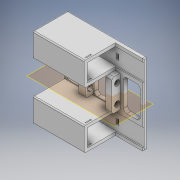
# Autodesk Inventor part: base_s
Saved by Autodesk Inventor 2020 (Build 240168000, 168)
## iProperties
Created: 2020-01-10
Part Number: base_s
Material: Generic
Document SubType Name: Modeling
Designer: Darien
Density: 1 g/cm^3
Appearance: Default
Author: Darien
Autodesk Inventor part; units mm, degrees
ref_plane "YZ Plane" through (0, 0, 0) normal (1, 0, 0) x (0, 1, 0)
ref_plane "XZ Plane" through (0, 0, 0) normal (0, 1, 0) x (-1, 0, 0)
sketch "Sketch1" plane through (0, 0, 0) normal (0, 0, 1) x (1, 0, 0)
  line L0 (-38.5, 45) -> (38.5, 45)
  line L1 (38.5, 45) -> (38.5, -45)
  line L2 (38.5, -45) -> (-38.5, -45)
  line L3 (-38.5, -45) -> (-38.5, 45)
  line L4 (-38.5, 45) -> (38.5, -45) construction
  line L5 (38.5, 45) -> (-38.5, -45) construction
  point P0 (0, 0)
  dimension "d0" = 90
  dimension "d1" = 77
  constraints: 12 end point, 2 midpoint, 2 parallel, 1 horizontal, 1 perpendicular
  measures "d0" distance of L1.end L0.end
  measures "d1" distance of L0.end L0.start
extrude "Extrusion1" add sketch "Sketch1" along normal blind 4
fillet "Fillet1" radius 4 4 edges at (-38.5, 45, 2) (-38.5, -45, 2) (38.5, 45, 2) (38.5, -45, 2)
sketch "Sketch15" plane through (0, 0, 4) normal (0, 0, 1) x (1, 0, 0)
  line L0 (34.5, 45) -> (-34.5, 45) construction
  line L1 (0, 45) -> (0, -45) construction
  line L2 (-34.5, -45) -> (34.5, -45) construction
  line L3 (-16, 15.4) -> (-10, 15.4)
  line L4 (-10, 15.4) -> (-10, -15)
  line L5 (-10, -15) -> (-16, -15)
  line L6 (-16, -15) -> (-16, 15.4)
  line L7 (-16, 15.4) -> (-10, -15) construction
  line L8 (-10, 15.4) -> (-16, -15) construction
  line L9 (16, 15.4) -> (10, 15.4)
  line L10 (10, 15.4) -> (10, -15)
  line L11 (10, -15) -> (16, -15)
  line L12 (16, -15) -> (16, 15.4)
  point P0 (-13, 0.2)
  dimension "d83" = 6
  dimension "d84" = 30.4
  dimension "d85" = 30
  dimension "d86" = 10
  constraints: 22 end point, 4 midpoint, 4 symmetric about line, 2 parallel, 1 horizontal, 1 perpendicular
  measures "d83" distance of L3.start L3.end
  measures "d84" distance of L5.end L3.start
  measures "d85" distance between parallel lines of L2 L5
  measures "d86" distance between parallel lines of L1 L4
extrude "Extrusion13" add sketch "Sketch15" along normal blind 7.8
sketch "Sketch16" plane through (16, -15.2, 4) normal (1, 0, 0) x (0, 0, -1)
  circle A0 centre (-2.75, 24.05) radius 2.65
  line L0 (-7.8, 0) -> (-7.8, 30.4) projected
  line L1 (0, 30.4) -> (-7.8, 30.4) projected
  line L2 (-7.8, 40.4) -> (-7.8, -10) construction
  line L3 (-7.8, 15.2) -> (0, 15.2) construction
  line L4 (0, -25.8) -> (0, 56.2) construction
  circle A1 centre (-2.75, 6.35) radius 2.65
  point P0 (4, 15.2)
  dimension "d62" = 5.05
  dimension "d63" = 6.35
  dimension "d64" = 5.3
  constraints: 2 centre point, 2 end point, 2 midpoint, 1 symmetric about line, 1 other
  measures "d62" distance from line of L0 A0.centre
  measures "d63" distance from line of L1 A0.centre
  measures "d64" diameter of A0
extrude "Extrusion14" cut sketch "Sketch16" against normal up to surface (32 mm away)
ref_plane "Work Plane2" through (17.25, -10.5, 0) normal (-1, 0, 0) x (0, 0, 1)
sketch "Sketch18" plane through (0, 0, 11.8) normal (0, 0, 1) x (1, 0, 0)
  line L0 (38.5, -41) -> (38.5, 41) projected
  line L1 (-38.5, -38.75) -> (38.5, -38.75)
  line L2 (38.5, -38.75) -> (38.5, 38.75)
  line L3 (38.5, 38.75) -> (-38.5, 38.75)
  line L4 (-38.5, 38.75) -> (-38.5, -38.75)
  line L5 (-38.5, -38.75) -> (38.5, 38.75) construction
  line L6 (38.5, -38.75) -> (-38.5, 38.75) construction
  line L7 (-38.5, -45.0251) -> (38.5, -45.0251)
  line L8 (38.5, -45.0251) -> (38.5, 45.0251)
  line L9 (38.5, 45.0251) -> (-38.5, 45.0251)
  line L10 (-38.5, 45.0251) -> (-38.5, -45.0251)
  line L11 (-38.5, -45.0251) -> (38.5, 45.0251) construction
  line L12 (38.5, -45.0251) -> (-38.5, 45.0251) construction
  point P0 (0, 0)
  point P1 (-38.5, 38.75)
  point P2 (-38.5, -38.75)
  dimension "d76" = 77.5
  constraints: 24 end point, 4 midpoint, 4 parallel, 2 horizontal, 2 perpendicular, 2 point on line
  measures "d76" distance between parallel lines of L3 L1
extrude "Extrusion16" cut sketch "Sketch18" against normal through all contours L8 L7 L10 L1 L0 | L3 L10 L9 L8 L0
sketch "Sketch19" plane through (10, -15, 4) normal (-1, 0, 0) x (0, 0, 1)
  circle A0 centre (2.75, 23.85) radius 2.65 projected
  circle A1 centre (2.75, 23.85) radius 3.2
  line L0 (0, 0) -> (0, 30.4) projected
  line L1 (0, 22.2137) -> (-0.0421, 25.4134)
  line L2 (-0.0421, 25.4134) -> (2.7079, 27.0497)
  line L3 (2.7079, 27.0497) -> (5.5, 25.4863)
  line L4 (5.5, 25.4863) -> (5.5421, 22.2866)
  line L5 (5.5421, 22.2866) -> (2.7921, 20.6503)
  line L6 (2.7921, 20.6503) -> (0, 22.2137)
  line L7 (0, 15.2) -> (7.8, 15.2)
  line L8 (7.8, 30.4) -> (7.8, 0) projected
  circle A2 centre (2.75, 6.55) radius 2.65
  circle A3 centre (2.75, 6.55) radius 3.2
  line L9 (0, 30.4) -> (0, 0.4)
  line L10 (-0.0421, 4.9866) -> (2.7079, 3.3503)
  line L11 (2.7079, 3.3503) -> (5.5, 4.9137)
  line L12 (5.5, 4.9137) -> (5.5421, 8.1134)
  line L13 (5.5421, 8.1134) -> (2.7921, 9.7497)
  line L14 (2.7921, 9.7497) -> (0, 8.1863)
  point P0 (-4, 15)
  point P1 (0, 30)
  point P2 (7.8, 30)
  point P3 (0, 8.1863)
  point P4 (0, 4.9615)
  point P5 (0, 25.4385)
  dimension "d87" = 6.4
  constraints: 26 end point, 10 symmetric about line, 3 coincident, 2 midpoint, 2 point on line, 1 centre point, 1 horizontal, 20 other
extrude "Extrusion17" cut sketch "Sketch19" along normal blind 23 and the other way blind 3 contours L14 L13 L12 L11 L10 L0 | L4 L5 L6 L0 L2 L3
fillet "Fillet3" radius 2 4 edges at (13, -15, 11.8) (-13, -15, 11.8) (13, 15.4, 11.8) (-13, 15.4, 11.8)
sketch "Sketch25" plane through (0, 0, 4) normal (0, 0, 1) x (1, 0, 0)
  line L0 (-38.5, -38.75) -> (38.5, -38.75) projected
  line L1 (38.5, -38.75) -> (38.5, 38.75) projected
  line L2 (-38.5, -38.75) -> (38.5, -38.75)
  line L3 (38.5, -38.75) -> (38.5, 38.75)
  line L4 (38.5, 38.75) -> (-38.5, 38.75)
  line L5 (-38.5, 38.75) -> (-38.5, -38.75)
  line L6 (-38.5, 38.75) -> (-38.5, -38.75) projected
  line L7 (-38.5, -38.75) -> (38.5, -38.75)
  line L8 (38.5, -38.75) -> (38.5, -15.75)
  line L9 (38.5, -15.75) -> (-38.5, -15.75)
  line L10 (-38.5, -15.75) -> (-38.5, -38.75)
  line L11 (-38.5, 38.75) -> (38.5, 38.75)
  line L12 (38.5, 38.75) -> (38.5, 15.75)
  line L13 (38.5, 15.75) -> (-38.5, 15.75)
  line L14 (-38.5, 15.75) -> (-38.5, 38.75)
  line L15 (11.5, -38.75) -> (11.5, -15.75)
  line L16 (11.5, 15.75) -> (11.5, 38.75)
  point P0 (0, 0)
  point P1 (38.5, -15.75)
  point P2 (-38.5, -15.75)
  dimension "d113" = 23
  dimension "d114" = 23
  dimension "d133" = 50
  dimension "d134" = 50
  constraints: 28 end point, 8 point on line, 6 parallel, 4 perpendicular, 3 horizontal
  measures "d113" distance between parallel lines of L9 L0
  measures "d114" distance between parallel lines of L4 L13
  measures "d133" distance between parallel lines of L10 L15
  measures "d134" distance between parallel lines of L5 L16
extrude "Extrusion23" add sketch "Sketch25" along normal blind 30 contours L5 L9 L15 L0 | L5 L4 L16 L13
sketch "Sketch26" plane through (38.5, -38.75, 0) normal (1, 0, 0) x (0, 0, -1)
  line L0 (-34, 77.5) -> (-34, 54.5) projected
  line L1 (0, 77.5) -> (0, 0) projected
  line L2 (-34, 77.5) -> (0, 77.5)
  line L3 (0, 77.5) -> (0, 54.5727)
  line L4 (0, 54.5727) -> (-34, 54.5727)
  line L5 (-34, 54.5727) -> (-34, 77.5)
  line L6 (-4, 23) -> (-34, 23) projected
  line L7 (0, 0) -> (-34, 0) projected
  line L8 (-34, 23) -> (0, 23)
  line L9 (0, 23) -> (0, 0)
  line L10 (0, 0) -> (-34, 0)
  line L11 (-34, 0) -> (-34, 23)
  line L12 (-31, 20) -> (-3, 20)
  line L13 (-3, 20) -> (-3, 3)
  line L14 (-3, 3) -> (-31, 3)
  line L15 (-31, 3) -> (-31, 20)
  line L16 (-31, 74.5) -> (-3, 74.5)
  line L17 (-3, 74.5) -> (-3, 57.5727)
  line L18 (-3, 57.5727) -> (-31, 57.5727)
  line L19 (-31, 57.5727) -> (-31, 74.5)
  point P0 (0, 38.75)
  dimension "d117" = 3
  dimension "d118" = 3
  constraints: 32 end point, 8 parallel, 4 perpendicular, 2 horizontal, 1 point on line, 6 other
  measures "d117" distance between parallel lines of L11 L15
  measures "d118" distance between parallel lines of L5 L19
extrude "Extrusion24" cut sketch "Sketch26" against normal blind 74 contours L12 L13 L14 L15 | L16 L17 L18 L19
fillet "Fillet6" radius 1 20 edges at (-13.5, -38.75, 34) (-38.5, -38.75, 17) (0, -38.75, 0) (-38.5, 0, 0) (38.5, 0, 0) (0, 38.75, 0) (38.5, 0.0364, 4) (38.5, 37.25, 4) (38.5, -37.25, 4) (38.5, -38.75, 2) (38.5, 38.75, 2) (-13.5, 15.75, 34) (-13.5, -15.75, 34) (-13.5, 38.75, 34) (-38.5, -27.25, 34) (-38.5, -15.75, 19) (-38.5, 27.25, 34) (-38.5, 38.75, 17) (-38.5, 15.75, 19) (-38.5, 0, 4)
sketch "Sketch27" plane through (0, 0, 4) normal (0, 0, 1) x (1, 0, 0)
  line L0 (-9, 15) -> (9, 15)
  line L1 (9, 15) -> (9, -15)
  line L2 (9, -15) -> (-9, -15)
  line L3 (-9, -15) -> (-9, 15)
  line L4 (-9, 15) -> (9, -15) construction
  line L5 (9, 15) -> (-9, -15) construction
  line L6 (-35.5, 15) -> (-19.5, 15)
  line L7 (-19.5, 15) -> (-19.5, -15)
  line L8 (-19.5, -15) -> (-35.5, -15)
  line L9 (-35.5, -15) -> (-35.5, 15)
  line L10 (-35.5, 15) -> (-19.5, -15) construction
  line L11 (-19.5, 15) -> (-35.5, -15) construction
  line L12 (-16, 13.4) -> (-16, -13) projected
  line L13 (19.5, 15) -> (35.5, 15)
  line L14 (35.5, 15) -> (35.5, -15)
  line L15 (35.5, -15) -> (19.5, -15)
  line L16 (19.5, -15) -> (19.5, 15)
  line L17 (19.5, 15) -> (35.5, -15) construction
  line L18 (35.5, 15) -> (19.5, -15) construction
  line L19 (16, -13) -> (16, 13.4) projected
  point P0 (0, 0)
  point P1 (-27.5, 0)
  point P2 (27.5, 0)
  dimension "d122" = 18
  dimension "d123" = 30
  dimension "d124" = 16
  dimension "d125" = 30
  dimension "d126" = 3.5
  dimension "d127" = 16
  dimension "d128" = 30
  dimension "d129" = 3.5
  constraints: 36 end point, 6 midpoint, 6 parallel, 3 horizontal, 3 perpendicular
  measures "d122" distance of L1.end L2.end
  measures "d123" distance of L0.end L1.end
  measures "d124" distance of L7.end L8.end
  measures "d125" distance of L6.end L7.end
  measures "d126" distance between parallel lines of L12 L7
  measures "d127" distance of L14.end L15.end
  measures "d128" distance of L13.end L14.end
  measures "d129" distance between parallel lines of L19 L16
extrude "Extrusion25" cut sketch "Sketch27" against normal up to surface (4 mm away)
fillet "Fillet7" radius 3 12 edges at (-19.5, 15, 2) (-35.5, 15, 2) (-35.5, -15, 2) (-19.5, -15, 2) (9, -15, 2) (35.5, -15, 2) (-9, -15, 2) (-9, 15, 2) (9, 15, 2) (19.5, 15, 2) (35.5, 15, 2) (19.5, -15, 2)
sketch "Sketch28" plane through (-35.5, 18.8227, 3) normal (0, 0, 1) x (1, 0, 0)
  line L0 (47, 0) -> (47, 16.9273) projected
  line L1 (47, 10.9273) -> (49.5, 10.9273)
  line L2 (49.5, 10.9273) -> (49.5, 5.9273)
  line L3 (49.5, 5.9273) -> (47, 5.9273)
  line L4 (47, 5.9273) -> (47, 10.9273)
  line L5 (73, 19.9273) -> (47, 19.9273) projected
  point P0 (35.5, -18.8227)
  point P1 (47, 5.9273)
  dimension "d135" = 5
  dimension "d136" = 2.5
  dimension "d137" = 9
  constraints: 8 end point, 2 parallel, 1 horizontal, 1 perpendicular, 1 point on line
  measures "d135" distance of L1.end L2.end
  measures "d136" distance of L2.end L3.end
  measures "d137" distance between parallel lines of L5 L1
extrude "Extrusion26" cut sketch "Sketch28" against normal through all
sketch "Sketch29" plane through (-37.5, 38.75, 1) normal (0, 1, 0) x (1, 0, 0)
  line L0 (47.6, -30) -> (46.6, -30)
  line L1 (46.6, -30) -> (46.6, -24.5)
  line L2 (46.6, -24.5) -> (47.6, -24.5)
  line L3 (47.6, -24.5) -> (47.6, -30)
  line L4 (49, -3) -> (49, -32) projected
  line L5 (0, -33) -> (49, -33) projected
  point P0 (37.5, 1)
  dimension "d140" = 1
  dimension "d141" = 5.5
  dimension "d142" = 1.4
  dimension "d143" = 3
  constraints: 8 end point, 2 parallel, 1 horizontal, 1 perpendicular
  measures "d140" distance of L0.start L0.end
  measures "d141" distance of L0.end L1.end
  measures "d142" distance between parallel lines of L4 L3
  measures "d143" distance between parallel lines of L5 L0
extrude "Extrusion27" cut sketch "Sketch29" against normal through all
ref_plane "Work Plane3" through (-37.5, 0, 1) normal (0, 1, 0) x (1, 0, 0)
mirror "Mirror2" about plane through (-37.5, 0, 1) normal (0, 1, 0) of "Extrusion26"
body "Solid1"
